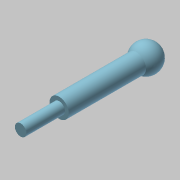
# Autodesk Inventor part: LinkPin
Saved by Autodesk Inventor 2015 (Build 190159000, 159)
## iProperties
Created: 2016-06-12
Part Number: LinkPin
Material: 一般
Document SubType Name: Modeling
Designer: kumagai
Density: 1 g/cm^3
Appearance: 既定
Author: kumagai
Autodesk Inventor part; units mm, degrees
ref_plane "YZ Plane" through (0, 0, 0) normal (1, 0, 0) x (0, 1, 0)
ref_plane "XZ Plane" through (0, 0, 0) normal (0, 1, 0) x (-1, 0, 0)
ref_plane "XY Plane" through (0, 0, 0) normal (0, 0, 1) x (1, 0, 0)
sketch "スケッチ1" plane through (0, 0, 0) normal (0, 0, 1) x (1, 0, 0)
  line L0 (0, 68.3935) -> (0, -34.7322) projected
  line L1 (-1.7907, 0) -> (10.7441, 0) projected
  line L2 (5, 40.101) -> (5, 0)
  line L3 (5, 0) -> (3, 0)
  line L4 (3, 0) -> (3, -20)
  line L5 (3, -20) -> (0, -20)
  arc A0 (5, 40.101) -> (0, 52) centre (0, 45) ccw
  line L6 (0, 52) -> (0, -20)
  point P0 (0, 0)
  dimension "d0" = 14
  dimension "d1" = 45
  dimension "d4" = 20
  dimension "d6" = 3
  dimension "d7" = 5
  constraints: 10 end point, 5 point on line, 2 perpendicular, 2 point on circle, 1 centre point, 1 vertical
  measures "d0" diameter of A0
  measures "d1" distance from line of L1 A0.centre
  measures "d4" distance from line of L4.end L1
  measures "d6" distance between parallel lines of L0 L4
  measures "d7" distance between parallel lines of L0 L2
revolve "回転1" add sketch "スケッチ1" angle 360 about axis through (0, 0, 0) along (0, -1, 0)
